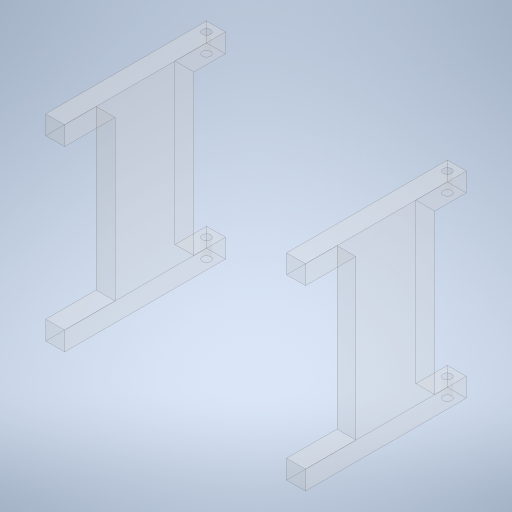
# Autodesk Inventor part: c
Saved by Autodesk Inventor 2024 (Build 280153000, 153)
## iProperties
Created: 2024-09-06
Part Number: c
Material: PMMA 플라스틱
Document SubType Name: Modeling
Designer: Eungang
Density: 1.188 g/cm^3
Appearance: 폴리카보네이트 - 선명
Mass: 27.638 g
Surface Area: 114.864 cm^2
Volume: 23.2643 cm^3
Author: Eungang
Autodesk Inventor part; units mm, degrees
ref_plane "YZ Plane" through (0, 0, 0) normal (1, 0, 0) x (0, 1, 0)
ref_plane "XZ Plane" through (0, 0, 0) normal (0, 1, 0) x (-1, 0, 0)
ref_plane "XY Plane" through (0, 0, 0) normal (0, 0, 1) x (1, 0, 0)
sketch "스케치1" plane through (0, 0, 0) normal (0, 0, 1) x (1, 0, 0)
  circle A0 centre (7.2, -7.2) radius 1.6 projected
  circle A1 centre (68.8, -7.2) radius 1.6 projected
  circle A2 centre (7.2, -48.8) radius 1.6 projected
  circle A3 centre (68.8, -48.8) radius 1.6 projected
  line L0 (73, -3) -> (3, -3) projected
  line L1 (3, -3) -> (3, -53) projected
  line L2 (3, -53) -> (73, -53) projected
  line L3 (73, -53) -> (73, -3) projected
  line L4 (22.5584, -24.5391) -> (23.3691, -24.5391) projected
  line L5 (23.3691, -24.5391) -> (23.3691, -29.9174) projected
  line L6 (23.3691, -29.9174) -> (25.4156, -29.9174) projected
  line L7 (25.4156, -29.9174) -> (25.4156, -30.6391) projected
  line L8 (25.4156, -30.6391) -> (20.5118, -30.6391) projected
  line L9 (20.5118, -30.6391) -> (20.5118, -29.9174) projected
  line L10 (20.5118, -29.9174) -> (22.5584, -29.9174) projected
  line L11 (22.5584, -29.9174) -> (22.5584, -24.5391) projected
  spline S0 degree 2 poles (29.6668, -24.9741) (29.9584, -24.6874) (30.7296, -24.4106) (31.2931, -24.4106) knots 0 0 0 1 2 2 2 projected
  spline S1 degree 2 poles (31.2931, -24.4106) (31.8319, -24.4106) (32.6328, -24.6924) (32.9145, -24.9741) knots 0 0 0 1 2 2 2 projected
  spline S2 degree 2 poles (32.9145, -24.9741) (33.2358, -25.2905) (33.4978, -26.1803) (33.4978, -26.8328) knots 0 0 0 1 2 2 2 projected
  line L12 (33.4978, -26.8328) -> (33.4978, -30.6391) projected
  line L13 (33.4978, -30.6391) -> (32.6871, -30.6391) projected
  line L14 (32.6871, -30.6391) -> (32.6871, -26.8328) projected
  spline S3 degree 2 poles (32.6871, -26.8328) (32.6871, -26.4077) (32.5784, -25.8343) (32.4251, -25.6019) knots 0 0 0 1 2 2 2 projected
  spline S4 degree 2 poles (32.4251, -25.6019) (32.262, -25.3548) (31.6985, -25.1027) (31.2931, -25.1027) knots 0 0 0 1 2 2 2 projected
  spline S5 degree 2 poles (31.2931, -25.1027) (30.9125, -25.1027) (30.3193, -25.3548) (30.1562, -25.6019) knots 0 0 0 1 2 2 2 projected
  spline S6 degree 2 poles (30.1562, -25.6019) (30.0029, -25.8343) (29.8942, -26.4028) (29.8942, -26.813) knots 0 0 0 1 2 2 2 projected
  line L15 (29.8942, -26.813) -> (29.8942, -30.6391) projected
  line L16 (29.8942, -30.6391) -> (29.0835, -30.6391) projected
  line L17 (29.0835, -30.6391) -> (29.0835, -26.8328) projected
  spline S7 degree 2 poles (29.0835, -26.8328) (29.0835, -26.1951) (29.3405, -25.2856) (29.6668, -24.9741) knots 0 0 0 1 2 2 2 projected
  line L18 (44.6696, -25.162) -> (44.6696, -24.5391) projected
  line L19 (44.6696, -24.5391) -> (47.0325, -24.5391) projected
  line L20 (47.0325, -24.5391) -> (47.0325, -25.162) projected
  line L21 (47.0325, -25.162) -> (46.2564, -25.162) projected
  line L22 (46.2564, -25.162) -> (46.2564, -30.0163) projected
  line L23 (46.2564, -30.0163) -> (47.0325, -30.0163) projected
  line L24 (47.0325, -30.0163) -> (47.0325, -30.6391) projected
  line L25 (47.0325, -30.6391) -> (44.6696, -30.6391) projected
  line L26 (44.6696, -30.6391) -> (44.6696, -30.0163) projected
  line L27 (44.6696, -30.0163) -> (45.4457, -30.0163) projected
  line L28 (45.4457, -30.0163) -> (45.4457, -25.162) projected
  line L29 (45.4457, -25.162) -> (44.6696, -25.162) projected
  spline S8 degree 2 poles (48.3623, -24.6083) (48.6292, -24.5194) (49.084, -24.4304) (49.4498, -24.4304) knots 0 0 0 1 2 2 2 projected
  spline S9 degree 2 poles (49.4498, -24.4304) (50.043, -24.4304) (51.0464, -24.8308) (51.4123, -25.2312) knots 0 0 0 1 2 2 2 projected
  spline S10 degree 2 poles (51.4123, -25.2312) (51.7781, -25.6267) (52.1785, -26.813) (52.1785, -27.5842) knots 0 0 0 1 2 2 2 projected
  spline S11 degree 2 poles (52.1785, -27.5842) (52.1785, -28.3504) (51.7879, -29.4874) (51.4172, -29.9075) knots 0 0 0 1 2 2 2 projected
  spline S12 degree 2 poles (51.4172, -29.9075) (51.0514, -30.3178) (50.0529, -30.7479) (49.4349, -30.7479) knots 0 0 0 1 2 2 2 projected
  spline S13 degree 2 poles (49.4349, -30.7479) (49.1285, -30.7479) (48.5896, -30.6589) (48.3623, -30.5897) knots 0 0 0 1 2 2 2 projected
  spline S14 degree 2 poles (48.3623, -30.5897) (48.1645, -30.5254) (47.7542, -30.3425) (47.5516, -30.2338) knots 0 0 0 1 2 2 2 projected
  line L30 (47.5516, -30.2338) -> (47.5516, -29.255) projected
  line L31 (47.5516, -29.255) -> (47.6158, -29.255) projected
  spline S15 degree 2 poles (47.6158, -29.255) (47.7246, -29.3539) (48.0607, -29.6307) (48.3029, -29.7642) knots 0 0 0 1 2 2 2 projected
  spline S16 degree 2 poles (48.3029, -29.7642) (48.5353, -29.8927) (49.084, -30.0558) (49.4399, -30.0558) knots 0 0 0 1 2 2 2 projected
  spline S17 degree 2 poles (49.4399, -30.0558) (49.8304, -30.0558) (50.5274, -29.7345) (50.7894, -29.428) knots 0 0 0 1 2 2 2 projected
  spline S18 degree 2 poles (50.7894, -29.428) (51.0464, -29.1166) (51.3332, -28.1724) (51.3332, -27.5842) knots 0 0 0 1 2 2 2 projected
  spline S19 degree 2 poles (51.3332, -27.5842) (51.3332, -26.9564) (51.0316, -26.0518) (50.7696, -25.7404) knots 0 0 0 1 2 2 2 projected
  spline S20 degree 2 poles (50.7696, -25.7404) (50.5126, -25.4388) (49.8255, -25.1323) (49.4399, -25.1323) knots 0 0 0 1 2 2 2 projected
  spline S21 degree 2 poles (49.4399, -25.1323) (49.0889, -25.1323) (48.4908, -25.3053) (48.2584, -25.4339) knots 0 0 0 1 2 2 2 projected
  spline S22 degree 2 poles (48.2584, -25.4339) (48.036, -25.5624) (47.7048, -25.8293) (47.6109, -25.9233) knots 0 0 0 1 2 2 2 projected
  line L32 (47.6109, -25.9233) -> (47.5516, -25.9233) projected
  line L33 (47.5516, -25.9233) -> (47.5516, -24.9544) projected
  spline S23 degree 2 poles (47.5516, -24.9544) (47.7542, -24.8604) (48.1101, -24.6874) (48.3623, -24.6083) knots 0 0 0 1 2 2 2 projected
  line L34 (41.1154, -27.1937) -> (38.9453, -24.5391) projected
  line L35 (38.9453, -24.5391) -> (39.9982, -24.5391) projected
  line L36 (39.9982, -24.5391) -> (41.9261, -26.9663) projected
  line L37 (41.9261, -26.9663) -> (42.8554, -26.9663) projected
  line L38 (42.8554, -26.9663) -> (42.8554, -24.5391) projected
  line L39 (42.8554, -24.5391) -> (43.6661, -24.5391) projected
  line L40 (43.6661, -24.5391) -> (43.6661, -30.6391) projected
  line L41 (43.6661, -30.6391) -> (42.0942, -30.6391) projected
  spline S24 degree 2 poles (42.0942, -30.6391) (41.5702, -30.6391) (40.8633, -30.5254) (40.542, -30.3178) knots 0 0 0 1 2 2 2 projected
  spline S25 degree 2 poles (40.542, -30.3178) (40.2207, -30.1102) (39.8499, -29.4626) (39.8499, -28.9831) knots 0 0 0 1 2 2 2 projected
  spline S26 degree 2 poles (39.8499, -28.9831) (39.8499, -28.3158) (40.5321, -27.4112) (41.1154, -27.1937) knots 0 0 0 1 2 2 2 projected
  spline S27 degree 2 poles (34.9907, -24.6083) (35.2576, -24.5194) (35.7124, -24.4304) (36.0782, -24.4304) knots 0 0 0 1 2 2 2 projected
  spline S28 degree 2 poles (36.0782, -24.4304) (36.6714, -24.4304) (37.6749, -24.8308) (38.0407, -25.2312) knots 0 0 0 1 2 2 2 projected
  spline S29 degree 2 poles (38.0407, -25.2312) (38.4065, -25.6267) (38.8069, -26.813) (38.8069, -27.5842) knots 0 0 0 1 2 2 2 projected
  spline S30 degree 2 poles (38.8069, -27.5842) (38.8069, -28.3504) (38.4164, -29.4874) (38.0456, -29.9075) knots 0 0 0 1 2 2 2 projected
  spline S31 degree 2 poles (38.0456, -29.9075) (37.6798, -30.3178) (36.6813, -30.7479) (36.0634, -30.7479) knots 0 0 0 1 2 2 2 projected
  spline S32 degree 2 poles (36.0634, -30.7479) (35.7569, -30.7479) (35.2181, -30.6589) (34.9907, -30.5897) knots 0 0 0 1 2 2 2 projected
  spline S33 degree 2 poles (34.9907, -30.5897) (34.793, -30.5254) (34.3827, -30.3425) (34.18, -30.2338) knots 0 0 0 1 2 2 2 projected
  line L42 (34.18, -30.2338) -> (34.18, -29.255) projected
  line L43 (34.18, -29.255) -> (34.2443, -29.255) projected
  spline S34 degree 2 poles (34.2443, -29.255) (34.353, -29.3539) (34.6892, -29.6307) (34.9314, -29.7642) knots 0 0 0 1 2 2 2 projected
  spline S35 degree 2 poles (34.9314, -29.7642) (35.1637, -29.8927) (35.7124, -30.0558) (36.0683, -30.0558) knots 0 0 0 1 2 2 2 projected
  spline S36 degree 2 poles (36.0683, -30.0558) (36.4588, -30.0558) (37.1558, -29.7345) (37.4178, -29.428) knots 0 0 0 1 2 2 2 projected
  spline S37 degree 2 poles (37.4178, -29.428) (37.6749, -29.1166) (37.9616, -28.1724) (37.9616, -27.5842) knots 0 0 0 1 2 2 2 projected
  spline S38 degree 2 poles (37.9616, -27.5842) (37.9616, -26.9564) (37.6601, -26.0518) (37.3981, -25.7404) knots 0 0 0 1 2 2 2 projected
  spline S39 degree 2 poles (37.3981, -25.7404) (37.141, -25.4388) (36.4539, -25.1323) (36.0683, -25.1323) knots 0 0 0 1 2 2 2 projected
  spline S40 degree 2 poles (36.0683, -25.1323) (35.7174, -25.1323) (35.1192, -25.3053) (34.8869, -25.4339) knots 0 0 0 1 2 2 2 projected
  spline S41 degree 2 poles (34.8869, -25.4339) (34.6644, -25.5624) (34.3332, -25.8293) (34.2393, -25.9233) knots 0 0 0 1 2 2 2 projected
  line L44 (34.2393, -25.9233) -> (34.18, -25.9233) projected
  line L45 (34.18, -25.9233) -> (34.18, -24.9544) projected
  spline S42 degree 2 poles (34.18, -24.9544) (34.3827, -24.8604) (34.7386, -24.6874) (34.9907, -24.6083) knots 0 0 0 1 2 2 2 projected
  line L46 (25.7962, -25.162) -> (25.7962, -24.5391) projected
  line L47 (25.7962, -24.5391) -> (28.1591, -24.5391) projected
  line L48 (28.1591, -24.5391) -> (28.1591, -25.162) projected
  line L49 (28.1591, -25.162) -> (27.383, -25.162) projected
  line L50 (27.383, -25.162) -> (27.383, -30.0163) projected
  line L51 (27.383, -30.0163) -> (28.1591, -30.0163) projected
  line L52 (28.1591, -30.0163) -> (28.1591, -30.6391) projected
  line L53 (28.1591, -30.6391) -> (25.7962, -30.6391) projected
  line L54 (25.7962, -30.6391) -> (25.7962, -30.0163) projected
  line L55 (25.7962, -30.0163) -> (26.5723, -30.0163) projected
  line L56 (26.5723, -30.0163) -> (26.5723, -25.162) projected
  line L57 (26.5723, -25.162) -> (25.7962, -25.162) projected
  line L58 (79.2, 3.2) -> (73.2, 3.2)
  line L59 (73.2, 3.2) -> (73.2, -2.8)
  line L60 (73.2, -2.8) -> (79.2, -2.8)
  line L61 (79.2, -2.8) -> (79.2, 3.2)
  line L62 (79.2, -59.2) -> (73.2, -59.2)
  line L63 (73.2, -59.2) -> (73.2, -53.2)
  line L64 (73.2, -53.2) -> (79.2, -53.2)
  line L65 (79.2, -53.2) -> (79.2, -59.2)
  line L66 (-3.2, 3.2) -> (2.8, 3.2)
  line L67 (2.8, 3.2) -> (2.8, -2.8)
  line L68 (2.8, -2.8) -> (-3.2, -2.8)
  line L69 (-3.2, -2.8) -> (-3.2, 3.2)
  line L70 (-3.2, -59.2) -> (2.8, -59.2)
  line L71 (2.8, -59.2) -> (2.8, -53.2)
  line L72 (2.8, -53.2) -> (-3.2, -53.2)
  line L73 (-3.2, -53.2) -> (-3.2, -59.2)
  line L74 (67.1, -22.175) -> (67.1, -28.175) projected
  line L75 (67.1, -28.175) -> (61.1, -28.175) projected
  line L76 (61.1, -28.175) -> (61.1, -22.175) projected
  line L77 (61.1, -22.175) -> (67.1, -22.175) projected
  circle A4 centre (7.2, -7.2) radius 1.6 projected
  circle A5 centre (68.8, -7.2) radius 1.6 projected
  circle A6 centre (7.2, -48.8) radius 1.6 projected
  circle A7 centre (68.8, -48.8) radius 1.6 projected
  line L78 (8.9, -22.175) -> (14.9, -22.175) projected
  line L79 (14.9, -22.175) -> (14.9, -28.175) projected
  line L80 (14.9, -28.175) -> (8.9, -28.175) projected
  line L81 (8.9, -28.175) -> (8.9, -22.175) projected
  line L82 (-3.2, -2.8) -> (-3.2, -53.2) projected
  line L83 (-3.2, -53.2) -> (2.8, -53.2) projected
  line L84 (2.8, -53.2) -> (2.8, -59.2) projected
  line L85 (2.8, -59.2) -> (73.2, -59.2) projected
  line L86 (73.2, -59.2) -> (73.2, -53.2) projected
  line L87 (73.2, -53.2) -> (79.2, -53.2) projected
  line L88 (79.2, -53.2) -> (79.2, -2.8) projected
  line L89 (79.2, -2.8) -> (73.2, -2.8) projected
  line L90 (73.2, -2.8) -> (73.2, 3.2) projected
  line L91 (73.2, 3.2) -> (2.8, 3.2) projected
  line L92 (2.8, 3.2) -> (2.8, -2.8) projected
  line L93 (2.8, -2.8) -> (-3.2, -2.8) projected
  point P0 (0, 0)
  dimension "d0" = 6
  dimension "d1" = 6
  dimension "d2" = 6
  dimension "d3" = 6
  dimension "d4" = 6
  dimension "d5" = 6
  dimension "d6" = 6
  dimension "d7" = 6
  constraints: 32 end point, 8 parallel, 4 horizontal, 4 perpendicular, 1 point on line
  measures "d0" distance of L60.end L59.end
  measures "d1" distance of L59.end L58.end
  measures "d2" distance of L63.end L64.end
  measures "d3" distance of L62.end L63.end
  measures "d4" distance of L67.end L68.end
  measures "d5" distance of L66.end L67.end
  measures "d6" distance of L72.end L71.end
  measures "d7" distance of L71.end L70.end
extrude "돌출1" add sketch "스케치1" along normal blind 45 contours L61 L60 L59 L58 | L67 L68 L69 L66 | L65 L62 L63 L64 | L72 L71 L70 L73
sketch "스케치2" plane through (79.2, -59.2, 0) normal (1, 0, 0) x (0, 0, -1)
  line L0 (-45, 0) -> (-45, 6) projected
  line L1 (-45, 6) -> (-51, 6) projected
  line L2 (-51, 0) -> (-51, 6) projected
  line L3 (-45, 0) -> (-51, 0) projected
  line L4 (-45, 56.4) -> (-45, 62.4) projected
  line L5 (-45, 62.4) -> (-51, 62.4) projected
  line L6 (-51, 56.4) -> (-51, 62.4) projected
  line L7 (-45, 56.4) -> (-51, 56.4) projected
  line L8 (6, 56.4) -> (6, 62.4) projected
  line L9 (6, 62.4) -> (0, 62.4) projected
  line L10 (0, 56.4) -> (0, 62.4) projected
  line L11 (6, 56.4) -> (0, 56.4) projected
  line L12 (6, 0) -> (6, 6) projected
  line L13 (6, 6) -> (0, 6) projected
  line L14 (0, 0) -> (0, 6) projected
  line L15 (6, 0) -> (0, 0) projected
  line L16 (0, 6) -> (0, 56.4) projected
  line L17 (-45, 6) -> (-45, 56.4) projected
  point P0 (0, 59.2)
extrude "돌출2" add sketch "스케치2" against normal blind 6
sketch "스케치3" plane through (-3.2, -2.8, 0) normal (-1, 0, 0) x (0, 0, 1)
  line L0 (45, 6) -> (45, 0) projected
  line L1 (45, 0) -> (51, 0) projected
  line L2 (51, 6) -> (51, 0) projected
  line L3 (45, 6) -> (51, 6) projected
  line L4 (45, -50.4) -> (45, -56.4) projected
  line L5 (45, -56.4) -> (51, -56.4) projected
  line L6 (51, -50.4) -> (51, -56.4) projected
  line L7 (45, -50.4) -> (51, -50.4) projected
  line L8 (-6, -50.4) -> (-6, -56.4) projected
  line L9 (-6, -56.4) -> (0, -56.4) projected
  line L10 (0, -50.4) -> (0, -56.4) projected
  line L11 (-6, -50.4) -> (0, -50.4) projected
  line L12 (-6, 6) -> (-6, 0) projected
  line L13 (-6, 0) -> (0, 0) projected
  line L14 (0, 6) -> (0, 0) projected
  line L15 (-6, 6) -> (0, 6) projected
  point P0 (0, 2.8)
extrude "돌출3" add sketch "스케치3" against normal blind 6
sketch "스케치4" plane through (-3.2, -2.8, 51) normal (-1, 0, 0) x (0, 0, 1)
  line L0 (-57, 0) -> (0, 0) projected
  line L1 (-57, -50.4) -> (0, -50.4) projected
  line L2 (-16, 0) -> (-41, 0)
  line L3 (-41, 0) -> (-41, -50.4)
  line L4 (-41, -50.4) -> (-16, -50.4)
  line L5 (-16, -50.4) -> (-16, 0)
  point P0 (-51, 2.8)
  point P1 (-16, -50.4)
  point P2 (-41, 0)
  constraints: 8 end point, 2 parallel, 2 point on line, 1 horizontal, 1 perpendicular
extrude "돌출4" add sketch "스케치4" against normal blind 6
sketch "스케치6" plane through (79.2, -59.2, 51) normal (1, 0, 0) x (0, 0, -1)
  line L0 (57, 6) -> (0, 6) projected
  line L1 (57, 56.4) -> (41, 56.4) projected
  line L2 (16, 6) -> (41, 6)
  line L3 (41, 6) -> (41, 56.4)
  line L4 (41, 56.4) -> (16, 56.4)
  line L5 (16, 56.4) -> (16, 6)
  point P0 (51, 59.2)
  point P1 (41, 6)
  constraints: 8 end point, 2 parallel, 1 horizontal, 1 perpendicular, 1 point on line
extrude "돌출5" add sketch "스케치6" against normal blind 6
sketch "스케치8" plane through (-3.2, -59.2, -6) normal (0, -1, 0) x (1, 0, 0)
  line L0 (0, 0) -> (0, 57) projected
  line L1 (6, 0) -> (6, 57) projected
  line L2 (0, 0) -> (6, 0)
  line L3 (6, 0) -> (6, 6)
  line L4 (6, 6) -> (0, 6)
  line L5 (0, 6) -> (0, 0)
  circle A0 centre (3, 3) radius 1.3
  line L6 (76.4, 0) -> (76.4, 57) projected
  line L7 (82.4, 0) -> (82.4, 57) projected
  line L8 (76.4, 0) -> (82.4, 0)
  line L9 (82.4, 0) -> (82.4, 6)
  line L10 (82.4, 6) -> (76.4, 6)
  line L11 (76.4, 6) -> (76.4, 0)
  circle A1 centre (79.4, 3) radius 1.3
  point P0 (3.2, 6)
  dimension "d18" = 2.6
  dimension "d19" = 2.6
  constraints: 16 end point, 4 parallel, 2 centre point, 2 horizontal, 2 perpendicular, 2 point on line
  measures "d18" diameter of A0
  measures "d19" diameter of A1
extrude "돌출6" cut sketch "스케치8" against normal up to next contours A0 | A1
sketch "스케치10" plane through (-3.2, -59.2, -6) normal (0, -1, 0) x (1, 0, 0)
  line L0 (0, 0) -> (0, 16) projected
  line L1 (6, 0) -> (6, 16) projected
  line L2 (0, 0) -> (6, 0)
  line L3 (6, 0) -> (6, 6)
  line L4 (6, 6) -> (0, 6)
  line L5 (0, 6) -> (0, 0)
  line L6 (82.4, 0) -> (76.4, 0) projected
  line L7 (82.4, 0) -> (82.4, 57) projected
  line L8 (76.4, 0) -> (82.4, 0)
  line L9 (82.4, 0) -> (82.4, 6)
  line L10 (82.4, 6) -> (76.4, 6)
  line L11 (76.4, 6) -> (76.4, 0)
  point P0 (3.2, 6)
  constraints: 16 end point, 4 parallel, 2 horizontal, 2 perpendicular, 2 point on line
extrude "돌출7" cut sketch "스케치10" against normal through all
sketch "스케치11" plane through (-3.2, -59.2, 51) normal (0, -1, 0) x (1, 0, 0)
  line L0 (0, -51) -> (0, 0) projected
  line L1 (6, -51) -> (6, -41) projected
  line L2 (0, -51) -> (6, -51)
  line L3 (6, -51) -> (6, -45)
  line L4 (6, -45) -> (0, -45)
  line L5 (0, -45) -> (0, -51)
  circle A0 centre (3, -48) radius 1.35
  line L6 (82.4, -51) -> (82.4, 0) projected
  line L7 (76.4, -51) -> (76.4, 0) projected
  line L8 (82.4, -51) -> (76.4, -51)
  line L9 (76.4, -51) -> (76.4, -45)
  line L10 (76.4, -45) -> (82.4, -45)
  line L11 (82.4, -45) -> (82.4, -51)
  circle A1 centre (79.4, -48) radius 1.35
  point P0 (3.2, -51)
  dimension "d24" = 2.7
  dimension "d25" = 2.7
  constraints: 16 end point, 4 parallel, 2 centre point, 2 horizontal, 2 perpendicular, 2 point on line
  measures "d24" diameter of A0
  measures "d25" diameter of A1
extrude "돌출8" cut sketch "스케치11" against normal through all contours A0 | A1
